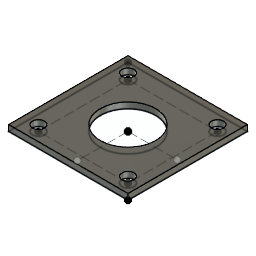
零部件1 (Autodesk Fusion 360 design; units mm, degrees)
Autodesk Fusion 360 part; units mm, degrees
sketch "草图1" plane through (0, 0, 5) normal (0, 0, 1) x (-1, 0, 0)
  line L0 (-20, 20) -> (-20, -20)
  line L1 (-20, -20) -> (20, -20)
  line L2 (20, -20) -> (20, 20)
  line L3 (20, 20) -> (-20, 20)
  circle A0 centre (0, 0) radius 9.25
  line L4 (0, 0) -> (-16.4715, 0) construction
  line L5 (0, 0) -> (0, 17) construction
  line L6 (-15, 15) -> (15, 15)
  line L7 (15, 15) -> (15, -15)
  line L8 (15, -15) -> (-15, -15)
  line L9 (-15, -15) -> (-15, 15)
  line L10 (-20, 20) -> (20, 20)
  line L11 (20, 20) -> (20, -20)
  line L12 (20, -20) -> (-20, -20)
  line L13 (-20, -20) -> (-20, 20)
  circle A1 centre (-15, -15) radius 2
  circle A2 centre (15, -15) radius 2
  circle A3 centre (15, 15) radius 2
  circle A4 centre (-15, 15) radius 2
  dimension "d1" = 18.5
  dimension "d2" = 30
  dimension "d3" = 30
  dimension "d4" = 4
  dimension "d5" = 4
  dimension "d6" = 4
  dimension "d7" = 4
  constraint coincident A0.centre L4.start
  constraint horizontal L4
  constraint perpendicular L4 L5
  constraint horizontal L6
  constraint vertical L7
  constraint horizontal L8
  constraint vertical L9
  constraint symmetric L5 L7 L9
  constraint symmetric L4 L6 L8
  constraint horizontal L10
  constraint vertical L11
  constraint horizontal L12
  constraint vertical L13
  constraint coincident L1.end L2.start
  constraint coincident L0.start L3.end
  constraint coincident L8.end L9.start
  constraint coincident L7.end L8.start
  constraint coincident L6.end L7.start
  constraint coincident L6.start L9.end
  measures "d1" diameter of A0
  measures "d2" distance of L6.end L7.end
  measures "d3" distance of L7 L9
  measures "d4" diameter of A1
  measures "d5" diameter of A2
  measures "d6" diameter of A3
  measures "d7" diameter of A4
extrude "拉伸1" add sketch "草图1" along normal blind 2 contours L0 L1 L2 L3 L10 L11 L12 L13 | A0 | L6 L9 A4 | L6 L9 A4 | L6 L7 L8 L9 A1 A2 A3 A4 | L6 L7 A3 | L6 L7 A3 | L8 L9 A1 | L8 L9 A1 | L7 L8 A2 | L7 L8 A2
extrude "拉伸2" cut sketch "草图1" along normal blind 5 contours A0 | L6 L9 A4 | L6 L9 A4 | L6 L7 A3 | L6 L7 A3 | L8 L9 A1 | L8 L9 A1 | L7 L8 A2 | L7 L8 A2
